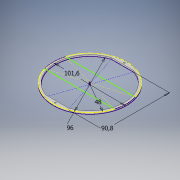
# Autodesk Inventor part: CortexHalter
Saved by Autodesk Inventor 2018 (Build 220112000, 112)
## iProperties
Created: 2017-06-10
Part Number: CortexHalter
Material: Generisch
Document SubType Name: Modeling
Designer: JochenAlt
Density: 1 g/cm^3
Appearance: Vorgabe
Author: JochenAlt
Autodesk Inventor part; units mm, degrees
ref_plane "YZ Plane" through (0, 0, 0) normal (1, 0, 0) x (0, 1, 0)
ref_plane "XZ Plane" through (0, 0, 0) normal (0, 1, 0) x (-1, 0, 0)
ref_plane "XY Plane" through (0, 0, 0) normal (0, 0, 1) x (1, 0, 0)
sketch "Skizze6" plane through (0, 0, 0) normal (0, 0, 1) x (1, 0, 0)
  circle A0 centre (0, 0) radius 50.8
  line L0 (15.5833, -45.4) -> (-15.5833, -45.4)
  line L1 (-15.5833, 45.4) -> (15.5833, 45.4)
  line L2 (15.5833, -45.4) -> (-15.5833, 45.4) construction
  line L3 (-15.5833, -45.4) -> (15.5833, 45.4) construction
  arc A1 (-15.5833, 45.4) -> (-15.5833, -45.4) centre (0, 0) ccw
  arc A2 (15.5833, -45.4) -> (15.5833, 45.4) centre (0, 0) ccw
  circle A3 centre (0, 0) radius 48 construction
  point P0 (0, -48)
  point P1 (0, 48)
  dimension "d40" = 101.6
  dimension "d42" = 90.8
  dimension "d45" = 48
  dimension "d46" = 96
  constraints: 8 end point, 6 point on circle, 4 centre point, 3 coincident, 2 midpoint, 1 horizontal, 1 parallel
  measures "d40" diameter of A0
  measures "d42" distance between parallel lines of L0 L1
  measures "d45" radius of A2
  measures "d46" diameter of A3
extrude "Extrusion3" add sketch "Skizze6" along normal blind 2
hole "Bohrung2" at (0, -48, 0) at (0, 48, 0) direction (0, 0, 1) diameter 2.1 end through all
sketch "Skizze7" plane through (0, 0, 2) normal (0, 0, 1) x (1, 0, 0)
  circle A0 centre (0, 0) radius 50.8 projected
  line L0 (48.6815, 14.5173) -> (-48.6815, 14.5173)
  line L1 (-48.6815, -14.5173) -> (48.6815, -14.5173)
  line L2 (48.6815, 14.5173) -> (-48.6815, -14.5173) construction
  line L3 (-48.6815, 14.5173) -> (48.6815, -14.5173) construction
  arc A1 (48.6815, -14.5173) -> (48.6815, 14.5173) centre (0, 0) ccw
  arc A2 (-48.6815, 14.5173) -> (-48.6815, -14.5173) centre (0, 0) ccw
  constraints: 8 end point, 5 point on circle, 2 centre point, 2 midpoint, 1 coincident, 1 horizontal, 1 parallel
